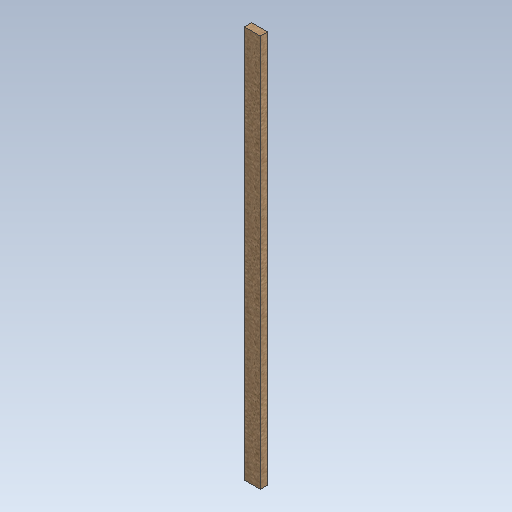
# Autodesk Inventor part: Separador Lateral
Saved by Autodesk Inventor 2020 (Build 240168000, 168)
## iProperties
Created: 2020-06-28
Part Number: Separador Lateral
Material: MDF Tablero de fibras de densidad media
Document SubType Name: Modeling
Designer: Pipi
Density: 0.8 g/cm^3
Appearance: Cartón - Ondulado
Author: Pipi
Autodesk Inventor part; units mm, degrees
ref_plane "YZ Plane" through (0, 0, 0) normal (1, 0, 0) x (0, 1, 0)
ref_plane "XZ Plane" through (0, 0, 0) normal (0, 1, 0) x (-1, 0, 0)
ref_plane "XY Plane" through (0, 0, 0) normal (0, 0, 1) x (1, 0, 0)
sketch "Boceto1" plane through (0, 0, 0) normal (0, 1, 0) x (-1, 0, 0)
  line L0 (11.3242, 29.6219) -> (11.3242, 24.1219)
  line L1 (11.3242, 24.1219) -> (-0.6758, 24.1219)
  line L2 (-0.6758, 24.1219) -> (-0.6758, 29.6219)
  line L3 (-0.6758, 29.6219) -> (11.3242, 29.6219)
  point P0 (0, 0)
  dimension "d0" = 5.5
  dimension "d1" = 12
  constraints: 8 end point, 3 perpendicular, 1 vertical
  measures "d0" distance of L0.start L0.end
  measures "d1" distance of L0.end L1.end
extrude "Extrusión1" add sketch "Boceto1" along normal blind 296.8
